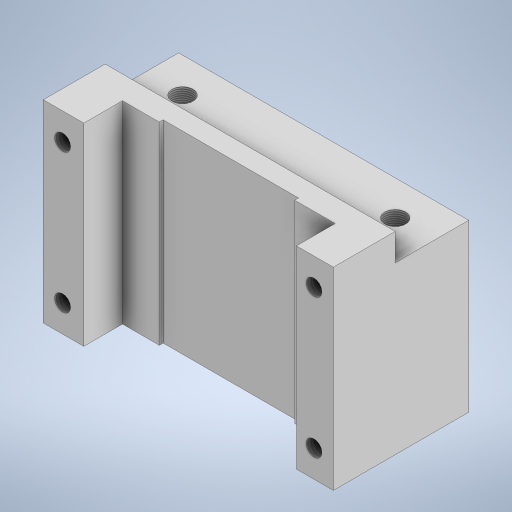
# Autodesk Inventor part: Lose Backe
Saved by Autodesk Inventor 2024 (Build 280153000, 153)
## iProperties
Created: 2023-05-10
Part Number: Lose Backe
Material: Generic
Document SubType Name: Modeling
Designer: dell
Density: 1 g/cm^3
Appearance: Default
Author: dell
Autodesk Inventor part; units mm, degrees
ref_plane "YZ Plane" through (0, 0, 0) normal (1, 0, 0) x (0, 1, 0)
ref_plane "XZ Plane" through (0, 0, 0) normal (0, 1, 0) x (-1, 0, 0)
ref_plane "XY Plane" through (0, 0, 0) normal (0, 0, 1) x (1, 0, 0)
sketch "Sketch1" plane through (0, 0, 0) normal (1, 0, 0) x (0, 1, 0)
  line L0 (-21.5, -17.5) -> (21.5, -17.5)
  line L1 (21.5, -17.5) -> (21.5, 1.5)
  line L2 (21.5, 17.5) -> (-21.5, 17.5)
  line L3 (-21.5, 17.5) -> (-21.5, -17.5)
  line L4 (-21.5, -17.5) -> (21.5, 17.5) construction
  line L5 (21.5, -17.5) -> (-21.5, 17.5) construction
  line L6 (18.0188, 17.5) -> (28.5, 17.5)
  line L7 (28.5, 17.5) -> (28.5, 1.5)
  line L8 (28.5, 1.5) -> (21.5, 1.5)
  point P0 (0, 0)
  dimension "d0" = 43
  dimension "d1" = 35
  dimension "d2" = 50
  dimension "d3" = 16
  constraints: 18 end point, 3 perpendicular, 2 horizontal, 2 midpoint, 2 parallel
  measures "d0" distance of L0.start L0.end
  measures "d1" distance of L0.end L2.start
  measures "d2" distance of L2.end L6.end
  measures "d3" distance of L6.end L7.end
extrude "Extrusion1" add sketch "Sketch1" along normal blind 75
sketch "Sketch2" plane through (0, 28.5, 17.5) normal (0, 1, 0) x (1, 0, 0)
  line L0 (0, 0) -> (75, 0) projected
  line L1 (65.4712, 0) -> (65.4712, 10)
  line L2 (65.4712, 10) -> (55, 10)
  line L3 (55, 10) -> (55, 11)
  line L4 (55, 11) -> (20, 11)
  line L5 (20, 11) -> (20, 10)
  line L6 (20, 10) -> (10.4712, 10)
  line L7 (10.4712, 10) -> (10.4712, 0)
  line L8 (0, 35) -> (75, 35) projected
  line L9 (37.5, 35) -> (37.5, 5.3668)
  point P0 (0, 17.5)
  dimension "d6" = 55
  dimension "d7" = 35
  dimension "d8" = 17.5
  dimension "d9" = 11
  dimension "d10" = 10
  constraints: 16 end point, 4 perpendicular, 4 point on line, 2 vertical, 1 horizontal, 1 midpoint
  measures "d6" distance between parallel lines of L7 L1
  measures "d7" distance between parallel lines of L5 L3
  measures "d8" distance between parallel lines of L5 L9
  measures "d9" distance between parallel lines of L0 L4
  measures "d10" distance between parallel lines of L0 L2
extrude "Extrusion2" cut sketch "Sketch2" against normal blind 75
sketch "Sketch6" plane through (0, -21.5, 17.5) normal (0, 0, 1) x (1, 0, 0)
  line L0 (0, 50) -> (0, 0) projected
  line L1 (0, 0) -> (10.4712, 0) projected
  point P0 (0, 21.5)
  point P1 (5, 7)
  dimension "d31" = 5
  dimension "d32" = 7
  measures "d31" distance from line of L0 point (5, 7)
  measures "d32" distance from line of point (5, 7) L1
hole "Hole1" at (5, -14.5, 17.5) direction (0, 0, -1) diameter 4.134 depth 14.2 tip angle 118 thread size "M5x0.8" class "6H" standard "ISO Metric profile"
pattern_linear "Rectangular Pattern1" count 2 spacing 36 along (0, 1, 0) count 2 spacing 65 along (1, 0, 0) of "Hole1"
sketch "Sketch8" plane through (0, -21.5, -17.5) normal (0, -1, 0) x (1, 0, 0)
  line L0 (0, 35) -> (0, 0) projected
  line L1 (0, 35) -> (10.4712, 35) projected
  point P0 (0, 17.5)
  point P1 (37.5, 11)
  dimension "d55" = 37.5
  dimension "d56" = 24
  measures "d55" distance from line of point (37.5, 11) L0
  measures "d56" distance from line of L1 point (37.5, 11)
hole "Hole3" at (37.5, -21.5, -6.5) direction (0, 1, 0) diameter 12 depth 20
sketch "Sketch9" plane through (0, -21.5, -17.5) normal (0, 0, -1) x (-1, 0, 0)
  line L0 (0, 0) -> (0, 43) projected
  line L1 (0, 0) -> (-75, 0) projected
  point P0 (0, 21.5)
  point P1 (-34, 7)
  dimension "d64" = 34
  dimension "d65" = 7
  measures "d64" distance from line of point (-34, 7) L0
  measures "d65" distance from line of L1 point (-34, 7)
hole "Hole4" at (34, -14.5, -17.5) direction (0, 0, 1) diameter 2.459 depth 8.8 thread size "M3x0.5" class "6H" standard "ISO Metric profile"
sketch "Sketch10" plane through (0, -21.5, -17.5) normal (0, -1, 0) x (1, 0, 0)
  line L0 (0, 35) -> (0, 0) projected
  line L1 (0, 35) -> (10.4712, 35) projected
  line L2 (65.4712, 35) -> (75, 35) projected
  point P0 (0, 17.5)
  point P1 (65, 9)
  point P2 (10, 9)
  dimension "d84" = 10
  dimension "d85" = 55
  dimension "d86" = 26
  dimension "d87" = 26
  measures "d84" distance from line of point (10, 9) L0
  measures "d85" distance of point (10, 9) point (65, 9)
  measures "d86" distance from line of L1 point (10, 9)
  measures "d87" distance from line of L2 point (65, 9)
hole "Hole6" at (65, -21.5, -8.5) at (10, -21.5, -8.5) direction (0, 1, 0) diameter 5.4587 end through all counterbore diameter 11 counterbore depth 7 thread size "M6x0.5" class "6H" standard "ISO Metric profile"
body "Solid1"
